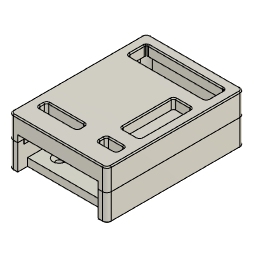
H743V2SnapMount (Autodesk Fusion 360 design; units mm, degrees)
Autodesk Fusion 360 part; units mm, degrees
note: some values were not read from the file. Set by a fixed rule: which face or edge a step refers to.
sketch "Wing Profile" plane through (0, 0, 0) normal (0, 0, 1) x (1, 0, 0) in component "Wing-V2"
  line L0 (-15.7, -27) -> (15.7, -27)
  line L1 (17.95, -24.75) -> (17.95, 24.75)
  line L2 (15.7, 27) -> (-15.7, 27)
  line L3 (-17.95, 24.75) -> (-17.95, -24.75)
  arc A0 (-15.7, 27) -> (-17.95, 24.75) centre (-15.7, 24.75) ccw
  arc A1 (17.95, 24.75) -> (15.7, 27) centre (15.7, 24.75) ccw
  arc A2 (15.7, -27) -> (17.95, -24.75) centre (15.7, -24.75) ccw
  arc A3 (-17.95, -24.75) -> (-15.7, -27) centre (-15.7, -24.75) ccw
  line L4 (0, 27) -> (0, -27) construction
  line L5 (18.45, -24.75) -> (18.45, 24.75)
  arc A4 (18.45, 24.75) -> (15.7, 27.5) centre (15.7, 24.75) ccw
  line L6 (15.7, 27.5) -> (-15.7, 27.5)
  arc A5 (-15.7, 27.5) -> (-18.45, 24.75) centre (-15.7, 24.75) ccw
  line L7 (-18.45, 24.75) -> (-18.45, -24.75)
  arc A6 (-18.45, -24.75) -> (-15.7, -27.5) centre (-15.7, -24.75) ccw
  line L8 (-15.7, -27.5) -> (15.7, -27.5)
  arc A7 (15.7, -27.5) -> (18.45, -24.75) centre (15.7, -24.75) ccw
  line L9 (-17.95, 0) -> (0, 0) construction
  line L10 (-17.95, 20) -> (-10.95, 20) construction
  line L11 (-10.95, 27) -> (-10.95, 20) construction
  line L12 (0, 2.5) -> (0, 20) construction
  line L13 (20, 0) -> (2.5, 0) construction
  line L14 (-16.95, 27) -> (16.95, 27)
  line L15 (17.95, 26) -> (17.95, 19.5)
  line L16 (16.95, 18.5) -> (-16.95, 18.5)
  line L17 (-17.95, 19.5) -> (-17.95, 26)
  arc A8 (-16.95, 27) -> (-17.95, 26) centre (-16.95, 26) ccw
  arc A9 (17.95, 26) -> (16.95, 27) centre (16.95, 26) ccw
  arc A10 (16.95, 18.5) -> (17.95, 19.5) centre (16.95, 19.5) ccw
  arc A11 (-17.95, 19.5) -> (-16.95, 18.5) centre (-16.95, 19.5) ccw
  line L18 (-16.95, -18.75) -> (-0.95, -18.75)
  line L19 (0.05, -19.75) -> (0.05, -21.75)
  line L20 (-0.95, -22.75) -> (-16.95, -22.75)
  line L21 (-17.95, -21.75) -> (-17.95, -19.75)
  arc A12 (-16.95, -18.75) -> (-17.95, -19.75) centre (-16.95, -19.75) ccw
  arc A13 (0.05, -19.75) -> (-0.95, -18.75) centre (-0.95, -19.75) ccw
  arc A14 (-0.95, -22.75) -> (0.05, -21.75) centre (-0.95, -21.75) ccw
  arc A15 (-17.95, -21.75) -> (-16.95, -22.75) centre (-16.95, -21.75) ccw
  line L22 (-8.95, -27) -> (-8.95, -22.75) construction
  line L23 (10.45, -18.75) -> (16.95, -18.75)
  line L24 (17.95, -19.75) -> (17.95, -21.75)
  line L25 (16.95, -22.75) -> (10.45, -22.75)
  line L26 (9.45, -21.75) -> (9.45, -19.75)
  arc A16 (17.95, -19.75) -> (16.95, -18.75) centre (16.95, -19.75) ccw
  arc A17 (16.95, -22.75) -> (17.95, -21.75) centre (16.95, -21.75) ccw
  arc A18 (9.45, -21.75) -> (10.45, -22.75) centre (10.45, -21.75) ccw
  arc A19 (10.45, -18.75) -> (9.45, -19.75) centre (10.45, -19.75) ccw
  line L27 (13.7, -22.75) -> (13.7, -27) construction
  line L28 (-20.45, 31.5) -> (20.45, 31.5)
  line L29 (22.45, 29.5) -> (22.45, -29.5)
  line L30 (20.45, -31.5) -> (-20.45, -31.5)
  line L31 (-22.45, -29.5) -> (-22.45, 29.5)
  arc A20 (22.45, 29.5) -> (20.45, 31.5) centre (20.45, 29.5) ccw
  arc A21 (20.45, -31.5) -> (22.45, -29.5) centre (20.45, -29.5) ccw
  arc A22 (-22.45, -29.5) -> (-20.45, -31.5) centre (-20.45, -29.5) ccw
  arc A23 (-20.45, 31.5) -> (-22.45, 29.5) centre (-20.45, 29.5) ccw
  line L32 (0, 31.5) -> (0, -31.5) construction
  line L33 (10.45, 12) -> (16.95, 12)
  line L34 (17.95, 11) -> (17.95, -11)
  line L35 (16.95, -12) -> (10.45, -12)
  line L36 (9.45, -11) -> (9.45, 11)
  arc A24 (10.45, 12) -> (9.45, 11) centre (10.45, 11) ccw
  arc A25 (17.95, 11) -> (16.95, 12) centre (16.95, 11) ccw
  arc A26 (16.95, -12) -> (17.95, -11) centre (16.95, -11) ccw
  arc A27 (9.45, -11) -> (10.45, -12) centre (10.45, -11) ccw
  line L37 (0, 0) -> (17.95, 0) construction
  line L38 (-15.7, -29.4) -> (15.7, -29.4)
  arc A28 (15.7, -29.4) -> (20.35, -24.75) centre (15.7, -24.75) ccw
  line L39 (20.35, -24.75) -> (20.35, 24.75)
  arc A29 (20.35, 24.75) -> (15.7, 29.4) centre (15.7, 24.75) ccw
  line L40 (15.7, 29.4) -> (-15.7, 29.4)
  arc A30 (-15.7, 29.4) -> (-20.35, 24.75) centre (-15.7, 24.75) ccw
  line L41 (-20.35, 24.75) -> (-20.35, -24.75)
  arc A31 (-20.35, -24.75) -> (-15.7, -29.4) centre (-15.7, -24.75) ccw
  line L42 (20.55, -24.75) -> (20.55, 24.75)
  arc A32 (20.55, 24.75) -> (15.7, 29.6) centre (15.7, 24.75) ccw
  line L43 (15.7, 29.6) -> (-15.7, 29.6)
  arc A33 (-15.7, 29.6) -> (-20.55, 24.75) centre (-15.7, 24.75) ccw
  line L44 (-20.55, 24.75) -> (-20.55, -24.75)
  arc A34 (-20.55, -24.75) -> (-15.7, -29.6) centre (-15.7, -24.75) ccw
  line L45 (-15.7, -29.6) -> (15.7, -29.6)
  arc A35 (15.7, -29.6) -> (20.55, -24.75) centre (15.7, -24.75) ccw
  point P0 (17.95, -27)
  point P1 (17.95, 27)
  point P2 (-17.95, 27)
  point P3 (-10.95, 20)
  point P4 (10.95, 20)
  point P5 (-10.95, -20)
  point P6 (10.95, -20)
  point P7 (-17.95, 27)
  point P8 (17.95, 27)
  point P9 (17.95, 18.5)
  point P10 (-17.95, -18.75)
  point P11 (0.05, -18.75)
  point P12 (0.05, -22.75)
  point P13 (9.45, -18.75)
  point P14 (17.95, -18.75)
  point P15 (17.95, -22.75)
  point P16 (-22.45, 31.5)
  point P17 (22.45, 31.5)
  point P18 (22.45, -31.5)
  point P19 (9.45, 12)
  point P20 (17.95, 12)
  point P21 (17.95, -12)
  constraint horizontal L0
  constraint vertical L1
  constraint horizontal L2
  constraint vertical L3
  constraint coincident P7 L3
  constraint coincident P7 L2
  constraint tangent L3 A0
  constraint tangent L2 A0
  constraint coincident P8 L2
  constraint coincident P8 L1
  constraint tangent L2 A1
  constraint tangent L1 A1
  constraint equal A0 A1
  constraint coincident P0 L1
  constraint coincident P0 L0
  constraint tangent L1 A2
  constraint tangent L0 A2
  constraint equal A0 A2
  constraint tangent L0 A3
  constraint tangent L3 A3
  constraint equal A0 A3
  constraint midpoint L2 L4.start
  constraint midpoint L0 L4.end
  constraint midpoint L9.end L4
  constraint midpoint L3 L9.start
  constraint coincident L9.end L37.start
  constraint horizontal L10
  constraint vertical L11
  constraint coincident P3 L10.end
  constraint coincident L2 L11.start
  constraint coincident L3 L10.start
  constraint symmetric P3 L12 P4
  constraint symmetric P3 L13 P5
  constraint symmetric P4 L13 P6
  constraint horizontal L14
  constraint vertical L15
  constraint horizontal L16
  constraint vertical L17
  constraint coincident P7 L14
  constraint coincident P7 L17
  constraint tangent L14 A8
  constraint tangent L17 A8
  constraint coincident P8 L14
  constraint coincident P8 L15
  constraint tangent L14 A9
  constraint tangent L15 A9
  constraint equal A8 A9
  constraint coincident P9 L15
  constraint coincident P9 L16
  constraint tangent L15 A10
  constraint tangent L16 A10
  constraint equal A8 A10
  constraint tangent L16 A11
  constraint tangent L17 A11
  constraint equal A8 A11
  constraint midpoint L4.start L14
  constraint horizontal L18
  constraint vertical L19
  constraint horizontal L20
  constraint vertical L21
  constraint coincident P10 L18
  constraint coincident P10 L21
  constraint tangent L18 A12
  constraint tangent L21 A12
  constraint coincident P11 L18
  constraint coincident P11 L19
  constraint tangent L18 A13
  constraint tangent L19 A13
  constraint equal A12 A13
  constraint coincident P12 L19
  constraint coincident P12 L20
  constraint tangent L19 A14
  constraint tangent L20 A14
  constraint equal A12 A14
  constraint tangent L20 A15
  constraint tangent L21 A15
  constraint equal A12 A15
  constraint collinear L3 L21
  constraint coincident L0 L22.start
  constraint coincident L20 L22.end
  constraint vertical L22
  constraint midpoint L20 L22.end
  constraint horizontal L23
  constraint vertical L24
  constraint horizontal L25
  constraint vertical L26
  constraint coincident P14 L23
  constraint coincident P14 L24
  constraint tangent L23 A16
  constraint tangent L24 A16
  constraint coincident P15 L24
  constraint coincident P15 L25
  constraint tangent L24 A17
  constraint tangent L25 A17
  constraint equal A16 A17
  constraint tangent L25 A18
  constraint tangent L26 A18
  constraint equal A16 A18
  constraint coincident P13 L23
  constraint coincident P13 L26
  constraint tangent L23 A19
  constraint tangent L26 A19
  constraint equal A16 A19
  constraint collinear L1 L24
  constraint midpoint L25 L27.start
  constraint coincident L0 L27.end
  constraint vertical L27
  constraint horizontal L28
  constraint vertical L29
  constraint horizontal L30
  constraint vertical L31
  constraint coincident P17 L28
  constraint coincident P17 L29
  constraint tangent L28 A20
  constraint tangent L29 A20
  constraint coincident P18 L29
  constraint coincident P18 L30
  constraint tangent L29 A21
  constraint tangent L30 A21
  constraint equal A20 A21
  constraint tangent L30 A22
  constraint tangent L31 A22
  constraint equal A20 A22
  constraint coincident P16 L28
  constraint coincident P16 L31
  constraint tangent L28 A23
  constraint tangent L31 A23
  constraint equal A20 A23
  constraint midpoint L28 L32.start
  constraint midpoint L30 L32.end
  constraint midpoint L9.end L32
  constraint horizontal L33
  constraint vertical L34
  constraint horizontal L35
  constraint vertical L36
  constraint coincident P19 L33
  constraint coincident P19 L36
  constraint tangent L33 A24
  constraint tangent L36 A24
  constraint coincident P20 L33
  constraint coincident P20 L34
  constraint tangent L33 A25
  constraint tangent L34 A25
  constraint equal A24 A25
  constraint coincident P21 L34
  constraint coincident P21 L35
  constraint tangent L34 A26
  constraint tangent L35 A26
  constraint equal A24 A26
  constraint tangent L35 A27
  constraint tangent L36 A27
  constraint equal A24 A27
  constraint midpoint L1 L37.end
  constraint midpoint L34 L37.end
  measures "d21" distance of P8 P7
  measures "d22" distance of P0 P8
  measures "d23" radius of A0
  measures "d112" distance of L10.start P3
  measures "d113" distance of L11.start P3
  measures "d137" distance of P7 P8
  measures "d138" distance of P8 P9
  measures "d139" radius of A8
  measures "d140" distance of P10 P11
  measures "d141" distance of P11 P12
  measures "d142" radius of A12
  measures "d143" distance of L22.start L22.end
  measures "d144" distance of P13 P14
  measures "d145" distance of P14 P15
  measures "d146" radius of A16
  measures "d147" distance of L27.start L27.end
  measures "d149" distance of P16 P17
  measures "d150" distance of P17 P18
  measures "d151" radius of A20
  measures "d161" distance of P19 P20
  measures "d162" distance of P20 P21
  measures "d163" radius of A24
extrude "Extrude Proxy" add sketch "Wing Profile" along normal blind 12.8 contours L0 L1 L3 A2 A3 L16 A10 A11 L18 L19 L20 A12 A13 A14 A15 L23 L25 L26 A16 A17 A18 A19 L33 L35 L36 A24 A25 A26 A27 | L3 L18 L19 L20 L21 A12 A13 A14 A15 | L1 L23 L24 L25 L26 A16 A17 A18 A19 | L1 L2 L3 A0 A1 L14 L15 L16 L17 A10 A11 | L1 L33 L34 L35 L36 A24 A25 A26 A27 makes body 1 in component "Wing-V2"
sketch "Wing Bottom Edge" plane through (0, -27, 0) normal (0, -1, 0) x (1, 0, 0) in component "Wing-V2"
  line L0 (0, 0) -> (5, 0) construction
  line L1 (5, 0) -> (5, 1.65) construction
  circle A0 centre (5, 1.65) radius 5.1
  line L2 (-18.45, 11.3) -> (18.45, 11.3)
  line L3 (18.45, 11.3) -> (18.45, -4)
  line L4 (18.45, -4) -> (-18.45, -4)
  line L5 (-18.45, -4) -> (-18.45, 11.3)
  line L6 (0, -4) -> (0, 0) construction
  line L7 (-18.45, 11.3) -> (18.45, 11.3)
  line L8 (18.45, 11.3) -> (18.45, 0)
  line L9 (18.45, 0) -> (-18.45, 0)
  line L10 (-18.45, 0) -> (-18.45, 11.3)
  dimension "d27" = 5
  dimension "d28" = 1.65
  dimension "d29" = 10.2
  dimension "d44" = 36.9
  dimension "d45" = 15.3
  dimension "d57" = 4
  dimension "d197" = 36.9
  dimension "d198" = 11.3
  constraint horizontal L0
  constraint vertical L1
  constraint coincident L0.start L6.end
  constraint coincident L1.end A0.centre
  constraint horizontal L2
  constraint vertical L3
  constraint horizontal L4
  constraint vertical L5
  constraint vertical L6
  constraint midpoint L4 L6.start
  constraint horizontal L7
  constraint vertical L8
  constraint horizontal L9
  constraint vertical L10
  constraint midpoint L0.start L9
  measures "d27" distance of L0.start L0.end
  measures "d28" distance of L0.end L1.end
  measures "d29" diameter of A0
  measures "d44" distance of L3.end L4.end
  measures "d45" distance of L2.end L3.end
  measures "d57" distance of L6.start L0.start
  measures "d197" distance of L8.end L9.end
  measures "d198" distance of L2.end L8.end
sketch "Wing Port Edge" plane through (-17.95, 0, 0) normal (-1, 0, 0) x (0, -1, 0) in component "Wing-V2"
  line L0 (-12.2, 12.8) -> (12.2, 12.8)
  line L1 (13.2, 11.8) -> (13.2, 2.65)
  line L2 (12.2, 1.65) -> (-12.2, 1.65)
  line L3 (-13.2, 2.65) -> (-13.2, 11.8)
  line L4 (0, 0) -> (0, 1.65)
  arc A0 (-12.2, 12.8) -> (-13.2, 11.8) centre (-12.2, 11.8) ccw
  arc A1 (13.2, 11.8) -> (12.2, 12.8) centre (12.2, 11.8) ccw
  arc A2 (12.2, 1.65) -> (13.2, 2.65) centre (12.2, 2.65) ccw
  arc A3 (-13.2, 2.65) -> (-12.2, 1.65) centre (-12.2, 2.65) ccw
  line L5 (-19, 6.15) -> (-19, 0) construction
  line L6 (-19, 0) -> (0, 0) construction
  line L7 (-23, 8.15) -> (-15, 8.15) construction
  line L8 (-15, 8.15) -> (-15, 6.15) construction
  line L9 (-15, 6.15) -> (-23, 6.15) construction
  line L10 (-23, 6.15) -> (-23, 8.15) construction
  line L11 (-23, 7.15) -> (-15, 7.15) construction
  line L12 (-15, 8.15) -> (-15, 6.15)
  line L13 (-15, 6.15) -> (-14, 6.15)
  line L14 (-14, 6.15) -> (-14, 8.15)
  line L15 (-14, 8.15) -> (-15, 8.15)
  line L16 (-23, 8.15) -> (-23, 6.15)
  line L17 (-23, 6.15) -> (-24, 6.15)
  line L18 (-24, 6.15) -> (-24, 8.15)
  line L19 (-24, 8.15) -> (-23, 8.15)
  point P0 (-13.2, 12.8)
  point P1 (13.2, 12.8)
  point P2 (13.2, 1.65)
  dimension "d35" = 26.4
  dimension "d36" = 11.15
  dimension "d37" = 1.65
  dimension "d39" = 1
  dimension "d218" = 6.15
  dimension "d222" = 19
  dimension "d223" = 8
  dimension "d224" = 2
  dimension "d225" = 1
  dimension "d226" = 1
  constraint horizontal L0
  constraint vertical L1
  constraint horizontal L2
  constraint vertical L3
  constraint vertical L4
  constraint coincident L4.start L6.end
  constraint coincident P0 L3
  constraint coincident P0 L0
  constraint tangent L3 A0
  constraint tangent L0 A0
  constraint coincident P1 L0
  constraint coincident P1 L1
  constraint tangent L0 A1
  constraint tangent L1 A1
  constraint equal A0 A1
  constraint coincident L2 L4.end
  constraint coincident P2 L1
  constraint coincident P2 L2
  constraint tangent L1 A2
  constraint tangent L2 A2
  constraint equal A0 A2
  constraint tangent L2 A3
  constraint tangent L3 A3
  constraint equal A0 A3
  constraint midpoint L2 L4.end
  constraint vertical L5
  constraint horizontal L6
  constraint coincident L5.end L6.start
  constraint horizontal L7
  constraint vertical L8
  constraint horizontal L9
  constraint vertical L10
  constraint midpoint L10 L11.start
  constraint midpoint L8 L11.end
  constraint midpoint L5.start L9
  constraint perpendicular L12 L13
  constraint parallel L12 L14
  constraint parallel L13 L15
  constraint perpendicular L16 L17
  constraint parallel L16 L18
  constraint parallel L17 L19
  measures "d35" distance of P0 P1
  measures "d36" distance of P1 P2
  measures "d37" distance of L4.start L4.end
  measures "d39" radius of A0
  measures "d218" distance of L5.start L5.end
  measures "d222" distance of L5.end L4.start
  measures "d223" distance of L7.start L7.end
  measures "d224" distance of L7.end L8.end
  measures "d225" distance of L8.end L13.end
  measures "d226" distance of L9.end L17.end
extrude "Extrude Cap" add sketch "Wing Bottom Edge" along normal blind 16 from surface at 3 separate body contours A0 L9 | A0 L9 makes body 2 in component "Wing-V2"
fillet "Filet Cap" radius 0.855 3 faces at (10.0966, -40.6667, 1.4633) (5.3888, -40.6667, 6.7352) (9.6425, -35.3333, -0.4613) on bodies 2 in component "Wing-V2"
extrude "Extrude Wire Base Cutter" add sketch "Wing Bottom Edge" along normal blind 4.5 separate body makes body 3 in component "Wing-V2"
extrude "Extrude Bottom Wire Cutter" add sketch "Wing Bottom Edge" along normal blind 4.5 and the other way blind 4.5 separate body contours A0 L9 | A0 L2 L3 L5 L7 L8 L9 L10 picked at (6.5148, 2.0295) makes body 4 in component "Wing-V2"
extrude "Extrude Port Cutter" add sketch "Wing Port Edge" along normal blind 4.5 separate body contours L0 L1 L2 L3 A0 A1 A2 A3 makes body 5 in component "Wing-V2"
extrude "Extrude Bottom" add sketch "Wing Profile" against normal blind 4 separate body contours L0 L1 L3 A2 A3 L16 A10 A11 L18 L19 L20 A12 A13 A14 A15 L23 L25 L26 A16 A17 A18 A19 L33 L35 L36 A24 A25 A26 A27 | L0 L1 L3 A2 A3 L5 A4 A5 L7 A6 L8 A7 L15 L17 A8 A9 L21 L24 L34 | L3 L18 L19 L20 L21 A12 A13 A14 A15 | L1 L23 L24 L25 L26 A16 A17 A18 A19 | L1 L2 L3 A0 A1 L14 L15 L16 L17 A10 A11 | L1 L33 L34 L35 L36 A24 A25 A26 A27 | A0 A5 L14 L17 A8 | L2 A4 L6 A5 L14 A8 A9 | A1 A4 L14 L15 A9 | A5 A8 | A4 A9 | L28 L29 L30 L31 A20 A21 A22 A23 | L38 A28 L39 A29 L40 A30 L41 A31 | L42 A32 L43 A33 L44 A34 L45 A35 makes body 6 in component "Mount"
extrude "Extrude Bottom Walls" add sketch "Wing Profile" along normal blind 6.15 separate body contours A5 A8 | A4 A9 | L28 L29 L30 L31 A20 A21 A22 A23 | L38 A28 L39 A29 L40 A30 L41 A31 | L42 A32 L43 A33 L44 A34 L45 A35 makes body 7 in component "Mount"
extrude "Extrude Bottom Overlap" add sketch "Wing Profile" along normal blind 2 from surface at 6.15 separate body contours L28 L29 L30 L31 A20 A21 A22 A23 makes body 8 in component "Mount"
extrude "Extrude Top Overlap" add sketch "Wing Profile" along normal blind 2 from surface at 6.15 separate body contours A5 A8 | A4 A9 | L38 A28 L39 A29 L40 A30 L41 A31 makes body 9 in component "Mount"
extrude "Extrude Top Walls" add sketch "Wing Profile" along normal blind 5.65 from surface at 8.15 separate body contours A5 A8 | A4 A9 | L28 L29 L30 L31 A20 A21 A22 A23 | L38 A28 L39 A29 L40 A30 L41 A31 | L42 A32 L43 A33 L44 A34 L45 A35 makes body 10 in component "Mount"
extrude "Extrude Top" add sketch "Wing Profile" along normal blind 4.5 from surface at 13.8 separate body contours L0 L1 L3 A2 A3 L16 A10 A11 L18 L19 L20 A12 A13 A14 A15 L23 L25 L26 A16 A17 A18 A19 L33 L35 L36 A24 A25 A26 A27 | L0 L1 L3 A2 A3 L5 A4 A5 L7 A6 L8 A7 L15 L17 A8 A9 L21 L24 L34 | L3 L18 L19 L20 L21 A12 A13 A14 A15 | L1 L23 L24 L25 L26 A16 A17 A18 A19 | L1 L2 L3 A0 A1 L14 L15 L16 L17 A10 A11 | L1 L33 L34 L35 L36 A24 A25 A26 A27 | A0 A5 L14 L17 A8 | L2 A4 L6 A5 L14 A8 A9 | A1 A4 L14 L15 A9 | A5 A8 | A4 A9 | L28 L29 L30 L31 A20 A21 A22 A23 | L38 A28 L39 A29 L40 A30 L41 A31 | L42 A32 L43 A33 L44 A34 L45 A35 makes body 11 in component "Mount"
combine "Join Bottom Walls" operation add target body 6 tool bodies 7 in component "Mount"
combine "Join Bottom Overlap" operation add target body 6 tool bodies 8 in component "Mount"
combine "Join Top Walls" operation add target body 11 tool bodies 10 in component "Mount"
combine "Join Top Overlap" operation add target body 11 tool bodies 9 in component "Mount"
combine "Cut Wires Top" operation cut target body 11 tool bodies 4 keep tools in component "Mount"
combine "Cut Wires Bottom" operation cut target body 6 tool bodies 3 in component "Mount"
extrude "Extrude Pin Cutter" add sketch "Wing Profile" along normal through all of body 11 from surface at 12.8 separate body contours L3 L18 L19 L20 L21 A12 A13 A14 A15 | L1 L23 L24 L25 L26 A16 A17 A18 A19 | L1 L2 L3 A0 A1 L14 L15 L16 L17 A10 A11 | L1 L33 L34 L35 L36 A24 A25 A26 A27 | A0 A5 L14 L17 A8 | A1 A4 L14 L15 A9 makes body 12 at (-11.6167, -18.75, 14.6333) makes body 13 at (12.6167, -18.75, 14.6333) makes body 14 at (-5.65, 21.3333, 12.8) makes body 15 at (15.1167, -3.6667, 12.8) in component "Wing-V2"
extrude "Extrude10" [no effect] in component "Mount"
combine "Cut Wires Wall" operation cut target body 6 tool bodies 4 in component "Mount"
combine "Cut Ports Bottom" operation cut target body 6 tool bodies 5 keep tools in component "Mount"
combine "Cut Ports Top" operation cut target body 11 tool bodies 5 in component "Mount"
combine "Cut Pins Top" operation cut target body 11 tool bodies 12 13 14 15 in component "Mount"
sketch "Tab" plane through (-20.35, 0, 0) normal (-1, 0, 0) x (0, -1, 0) in component "Mount"
  line L0 (-15, 6.15) -> (-14, 6.15)
  line L1 (-23, 8.15) -> (-23, 6.15)
  line L2 (-23, 8.15) -> (-15, 8.15) construction
  line L3 (-15, 6.15) -> (-23, 6.15) construction
  line L4 (-23, 7.15) -> (-15, 7.15) construction
  line L5 (-19, 6.15) -> (-19, 0) construction
  line L6 (-24, 8.15) -> (-23, 8.15)
  line L7 (-15, 8.15) -> (-15, 6.15)
  line L8 (-23, 6.15) -> (-24, 6.15)
  line L9 (-24, 6.15) -> (-24, 8.15)
  line L10 (-23, 6.15) -> (-23, 8.15) construction
  line L11 (-14, 8.15) -> (-15, 8.15)
  line L12 (-15, 8.15) -> (-15, 6.15) construction
  line L13 (-14, 6.15) -> (-14, 8.15)
  line L14 (-19, 0) -> (0, 0) construction
  dimension "d230" = 6.15
  dimension "d231" = 19
  dimension "d232" = 8
  dimension "d233" = 2
  dimension "d234" = 1
  dimension "d235" = 1
  constraint vertical L5
  constraint horizontal L14
  constraint coincident L5.end L14.start
  constraint horizontal L2
  constraint vertical L12
  constraint horizontal L3
  constraint vertical L10
  constraint midpoint L4.start L10
  constraint midpoint L4.end L12
  constraint midpoint L5.start L3
  constraint perpendicular L0 L7
  constraint parallel L7 L13
  constraint parallel L0 L11
  constraint perpendicular L1 L8
  constraint parallel L1 L9
  constraint parallel L6 L8
  constraint coincident L14.end origin
  measures "d230" distance of L5.start L5.end
  measures "d231" distance of L5.end L14.end
  measures "d232" distance of L1.start L2.end
  measures "d233" distance of L0.start L2.end
  measures "d234" distance of L0.end L0.start
  measures "d235" distance of L8.end L1.end
ref_plane "WorkPlane2" through (-20.35, 19, 7.15) normal (0, -1, 0) x (1, 0, 0) in component "Mount"
sketch "Snap" plane through (-20.35, 19, 7.15) normal (0, -1, 0) x (1, 0, 0) in component "Mount"
  circle A0 centre (0, -0.375) radius 0.625
  line L0 (0, -1) -> (0, 1)
  line L1 (0, -1) -> (1.9, -1)
  point P0 (0, -1)
  dimension "d238" = 1.25
  constraint coincident A0.centre L0
  constraint tangent A0 L1
  measures "d238" diameter of A0
extrude "Extrude Snap" add sketch "Snap" along normal mid plane 8 contours A0 L0 picked at (-0.1629, -0.5049) bodies 11 in component "Mount"
mirror "Mirror Snap FB" about plane through (0, 0, 0) normal (0, 1, 0) of "Extrude Snap" in component "Mount"
mirror "Mirror Snap LR" about plane through (0, 0, 0) normal (1, 0, 0) of "Extrude Snap", "Mirror Snap FB" in component "Mount"
combine "Cut Snaps" operation cut target body 6 tool bodies 11 keep tools in component "Mount"
ref_plane "WorkPlane3" through (0, 31.5, 8.15) normal (1, 0, 0) x (0, 1, 0) in component "Mount"
sketch "Grab" plane through (0, 31.5, 8.15) normal (1, 0, 0) x (0, 1, 0) in component "Mount"
  circle A0 centre (0, 1.25) radius 1.25
  line L0 (0, 0) -> (0, 10.15)
  line L1 (-2, 0) -> (0, 0)
  dimension "d246" = 2.5
  constraint coincident A0.centre L0
  constraint tangent A0 L1
  measures "d246" diameter of A0
extrude "Extrude Grab" add sketch "Grab" along normal mid plane 28 contours A0 L0 picked at (0.2729, 1.5649) bodies 11 in component "Mount"
fillet "Filet Mount" radius 0.5 2 faces at (-6.15, 10.6667, -4) (-2.8167, 3.5833, 18.3) on bodies 6 11 in component "Mount"
hole "Cut Screw Holes" at (-10.95, 20, 0) at (10.95, 20, 0) at (10.95, -20, 0) at (-10.95, -20, 0) direction (0, 0, -1) diameter 2.8448 depth 4 tip angle 180 countersink diameter 5.715 countersink angle 82 bodies 6 in component "Mount"
component "Wing-V2" placed x (1, 0, 0) y (0, 1, 0) z (0, 0, 1) at (0, 0, 0)
component "Mount" placed x (1, 0, 0) y (0, 1, 0) z (0, 0, 1) at (0, 0, 0)
equation "WingWidth = 35.9 mm" comment "Width of all 3 circuit boards"
equation "WingLegnth = 54 mm" comment "Length of the bottom circuit board"
equation "WingBottomHeight = 1.65 mm" comment "Height of the bottom circuit board"
equation "WingBottomToTop = 12.8 mm" comment "From bottom of board to top of board"
equation "CapDiameter = 10.2 mm" comment "Diameter of the capacitor"
equation "CapHeight = 16 mm" comment "Height of the capacitor"
equation "CapBottomOffset = 3 mm" comment "Offset between bottom of board and capacitor"
equation "WingPortWidth = 26.4 mm" comment "Width of the port area including SD"
equation "WingBoardRadius = 2.25 mm" comment "Radius of the board filet"
equation "d21 = WingWidth"
equation "d22 = WingLegnth"
equation "d23 = WingBoardRadius"
equation "d24 = WingBottomToTop"
equation "WingBottomCenterToCap = 5 mm" comment "Offset from center to cap"
equation "d27 = WingBottomCenterToCap"
equation "d28 = WingBottomHeight"
equation "d29 = CapDiameter"
equation "d30 = CapBottomOffset"
equation "d31 = CapHeight"
equation "d35 = WingPortWidth"
equation "d36 = WingBottomToTop - WingBottomHeight"
equation "d37 = WingBottomHeight"
equation "WingPortFiletRadius = 1.0 mm"
equation "d39 = WingPortFiletRadius"
equation "WallThickness = 4 mm" comment "How thick the walls are"
equation "InnerGap = 0.5 mm" comment "Gap between Wing and Wall"
equation "d42 = InnerGap + WallThickness"
equation "d44 = WingWidth + WireGap"
equation "d45 = TotalHeight - TopHeight - TopWireOverhang"
equation "d49 = InnerGap"
equation "SplitHeight = TotalHeight / 2" comment "The height at where the top and bottom are split"
equation "BottomHeight = 4 mm" comment "Height of the base"
equation "d53 = -BottomHeight"
equation "d55 = BottomWallHeight"
equation "d57 = BottomHeight"
equation "WireGap = 1 mm" comment "Extra gap around wire area"
equation "d61 = InnerGap + WallThickness"
equation "MountFiletRadius = 0.5 mm"
equation "MountHoleOffset = 7 mm" comment "Offset between board edge and mount hole"
equation "d112 = MountHoleOffset"
equation "d113 = MountHoleOffset"
equation "ScrewHeadHeight = 0.68 in" comment "Head heighg for #4 screw"
equation "ScrewHeadDiameter = 0.225 in" comment "Head diameter for #4 screw"
equation "ScrewShankDiameter = 0.112 in" comment "Shank diameter for #4 screw"
equation "d122 = BottomHeight"
equation "d123 = ScrewShankDiameter"
equation "d125 = ScrewHeadDiameter"
equation "d126 = ScrewHeadAngle"
equation "ScrewHeadAngle = 82 deg" comment "Head angle of #4 screw"
equation "PinsBackLength = 8.5 mm" comment "Length of the hole for the back pins header"
equation "PinsRightWidth = 8.5 mm" comment "With of hole for the right pins header"
equation "PinsRightLength = 24 mm" comment "Length of the hole for the right pins header"
equation "PinsFrontLength = 4 mm" comment "Length of the hole for the front pins"
equation "PinsFrontLeftWidth = 18 mm" comment "Width of the hoe for the front-left pins"
equation "PinsFrontRightWidth = 8.5 mm" comment "Width of the hole for the front-right pins"
equation "PinsFrontOffset = 4.25 mm" comment "Offset from front of the top board to the front holes"
equation "PinsHoleRadius = 1 mm" comment "Radus of the cut holes for the pins"
equation "TopHeight = 4.5 mm" comment "Height of the top cover"
equation "d137 = WingWidth"
equation "d138 = PinsBackLength"
equation "d139 = PinsHoleRadius"
equation "d140 = PinsFrontLeftWidth"
equation "d141 = PinsFrontLength"
equation "d142 = PinsHoleRadius"
equation "d143 = PinsFrontOffset"
equation "d144 = PinsFrontRightWidth"
equation "d145 = PinsFrontLength"
equation "d146 = PinsHoleRadius"
equation "d147 = PinsFrontOffset"
equation "OuterRadius = 2 mm" comment "The outside radius of the case."
equation "d149 = WingWidth + ( InnerGap * 2 ) + ( WallThickness * 2 )"
equation "d150 = WingLegnth + ( InnerGap * 2 ) + ( WallThickness * 2 )"
equation "d151 = OuterRadius"
equation "d152 = BottomWallHeight + WallOverlap + TopWallHeight"
equation "d153 = TopHeight"
equation "d155 = BottomWallHeight + WallOverlap"
equation "d156 = TopWallHeight"
equation "d158 = WingBottomToTop"
equation "d161 = PinsRightWidth"
equation "d162 = PinsRightLength"
equation "d163 = PinsHoleRadius"
equation "TopWireOverhang = 2 mm" comment "How much the top hangs over the wire port on the front edge."
equation "LatchSplitOffset = 4 mm" comment "The distance from the split to the base of the latch"
equation "d196 = MountFiletRadius"
equation "d197 = WingWidth + WireGap"
equation "d198 = TotalHeight - BottomHeight - TopHeight - TopWireOverhang"
equation "d199 = InnerGap + WallThickness"
equation "d201 = InnerGap + WallThickness"
equation "SnapDiameter = 1.25 mm" comment "Diameter of the snap components"
equation "GrabDiameter = 2.5 mm" comment "Diameter of the grab rails"
equation "WallOverlap = 2 mm" comment "The total amount that the walls overlap"
equation "TotalHeight = WingBottomToTop + BottomHeight + TopHeight + InnerGap" comment "Total height of the entire mount"
equation "WallOverlapGap = 0.2 mm" comment "The gap between the top and bottom walls"
equation "d208 = ( InnerGap + ( WallThickness / 2 ) ) - ( WallOverlapGap / 2 )"
equation "d209 = ( InnerGap + ( WallThickness / 2 ) ) + ( WallOverlapGap / 2 )"
equation "d210 = BottomWallHeight"
equation "d211 = WallOverlap"
equation "TopWallHeight = SplitHeight - TopHeight - ( WallOverlap / 2 ) + ( InnerGap / 2 )" comment "Height of top walls"
equation "BottomWallHeight = SplitHeight - BottomHeight - ( WallOverlap / 2 ) + ( InnerGap / 2 )"
equation "d215 = BottomWallHeight"
equation "d216 = WallOverlap"
equation "d218 = BottomWallHeight"
equation "TabWidth = 8 mm" comment "Width of the compression tabs in the lid."
equation "TabNotchWidth = 1 mm" comment "The cut that separates the tab from the overlap."
equation "TabCenterOffset = 19 mm" comment "Distance from center of mount to center of tabs."
equation "d222 = TabCenterOffset"
equation "d223 = TabWidth"
equation "d224 = WallOverlap"
equation "d225 = TabNotchWidth"
equation "d226 = TabNotchWidth"
equation "d230 = BottomWallHeight"
equation "d231 = TabCenterOffset"
equation "d232 = TabWidth"
equation "d233 = WallOverlap"
equation "d234 = TabNotchWidth"
equation "d235 = TabNotchWidth"
equation "d238 = SnapDiameter"
equation "d239 = TabWidth / 2"
equation "d246 = GrabDiameter"
equation "GrabWidth = 28 mm" comment "Width of grab handles"
equation "d248 = GrabWidth / 2"
equation "d250 = WingBottomToTop"
named bodies: "Wing Proxy", "Capacitor", "Port Cutter", "Bottom", "Bottom Walls", "Bottom Wire Cutter", "Top", "Top Walls", "Wall Wire Cutter", "Bottom Wall Overlap", "Top Wall Overlap"
